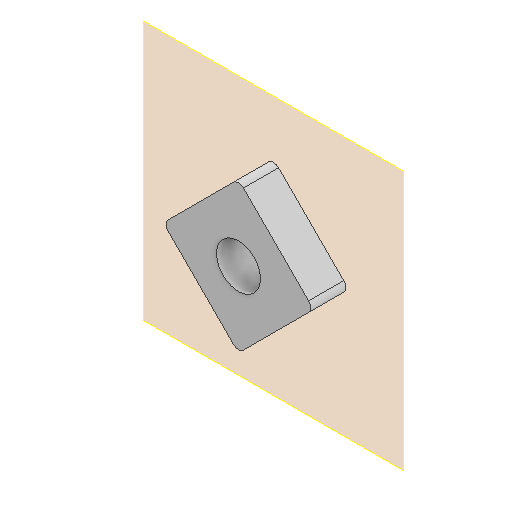
# Autodesk Inventor part: IM_Matchboxscope_lightdiffusor
Saved by Autodesk Inventor 2022 (Build 260153000, 153)
## iProperties
Created: 2023-06-16
Part Number: IM_Matchboxscope_lightdiffusor
Material: Generisch
Document SubType Name: Modeling
Designer: diederichbenedict
Density: 1 g/cm^3
Appearance: Vorgabe
Author: diederichbenedict
Autodesk Inventor part; units mm, degrees
ref_plane "YZ Plane" through (0, 0, 0) normal (1, 0, 0) x (0, 1, 0)
ref_plane "XZ Plane" through (0, 0, 0) normal (0, 1, 0) x (-1, 0, 0)
ref_plane "XY Plane" through (0, 0, 0) normal (0, 0, 1) x (1, 0, 0)
ref_plane "Arbeitsebene1" through (0, 0, 0) normal (0, 0, 1) x (1, 0, 0)
sketch "Skizze1" plane through (0, 0, 0) normal (0, 0, 1) x (1, 0, 0)
  circle A0 centre (-5.0971, -17.293) radius 1.4
  circle A1 centre (-17.4192, -5.2278) radius 1.4
  arc A2 (5.6957, 26.2674) -> (7.9686, 25.6694) centre (6.0612, 23.038) ccw
  arc A3 (5.6957, 26.2674) -> (-18.8161, -19.193) centre (0, 0) ccw
  arc A4 (-18.1702, -19.8055) -> (-18.8161, -19.193) centre (-16.2778, -17.1634) ccw
  arc A5 (-18.1702, -19.8055) -> (25.9554, 6.9811) centre (0, 0) ccw
  arc A6 (25.2463, 9.2218) -> (25.9554, 6.9811) centre (22.7119, 7.1872) ccw
  arc A7 (25.2463, 9.2218) -> (7.9686, 25.6694) centre (0, 0) ccw
  spline S0 degree 3 poles (-11.5553, -6.2972) (-11.3711, -6.4814) (-11.2247, -6.6998) (-11.0238, -7.1803) (-10.9713, -7.4379) (-10.9679, -7.9586) (-11.0171, -8.2168) (-11.2083, -8.6915) (-11.3454, -8.905) (-11.5184, -9.0874) knots 0 0 0 0 0.252225 0.252225 0.504373 0.504373 0.756494 0.756494 1 1 1 1
  line L0 (-11.5553, -6.2972) -> (-16.3497, -1.5028)
  arc A8 (-16.3497, 1.4985) -> (-16.3497, -1.5028) centre (-14.8491, -0.0022) ccw
  line L1 (-16.3497, 1.4985) -> (-1.5005, 16.3477)
  arc A9 (1.5007, 16.3477) -> (-1.5005, 16.3477) centre (0.0001, 14.8471) ccw
  line L2 (1.5007, 16.3477) -> (16.35, 1.4985)
  arc A10 (16.35, -1.5028) -> (16.35, 1.4985) centre (14.8494, -0.0022) ccw
  line L3 (16.35, -1.5028) -> (1.5007, -16.352)
  arc A11 (-1.5005, -16.352) -> (1.5007, -16.352) centre (0.0001, -14.8514) ccw
  line L4 (-1.5005, -16.352) -> (-4.7949, -13.0576)
  spline S1 degree 3 poles (-7.585, -13.0208) (-7.3961, -12.8415) (-7.1739, -12.7009) (-6.6882, -12.5128) (-6.4293, -12.4671) (-5.9087, -12.4775) (-5.6519, -12.5335) (-5.1824, -12.7372) (-4.9727, -12.8798) (-4.7949, -13.0576) knots 0 0 0 0 0.252231 0.252231 0.504388 0.504388 0.756517 0.756517 1 1 1 1
  arc A12 (-11.5184, -9.0874) -> (-7.585, -13.0208) centre (-9.4998, -11.0022) ccw
  line L5 (-4.7949, -13.0576) -> (-11.5553, -6.2972)
  line L6 (-15.9962, -1.1492) -> (-11.2017, -5.9437)
  arc A13 (-11.1557, -9.4315) -> (-7.9291, -12.658) centre (-9.4998, -11.0022) ccw
  line L7 (-4.4413, -12.7041) -> (-1.1469, -15.9985)
  arc A14 (-1.1469, -15.9985) -> (1.1472, -15.9985) centre (0.0001, -14.8514) ccw
  line L8 (1.1472, -15.9985) -> (15.9964, -1.1492)
  arc A15 (15.9964, -1.1492) -> (15.9964, 1.1449) centre (14.8494, -0.0022) ccw
  line L9 (15.9964, 1.1449) -> (1.1472, 15.9941)
  arc A16 (1.1472, 15.9941) -> (-1.1469, 15.9941) centre (0.0001, 14.8471) ccw
  line L10 (-1.1469, 15.9941) -> (-15.9962, 1.1449)
  arc A17 (-15.9962, 1.1449) -> (-15.9962, -1.1492) centre (-14.8491, -0.0022) ccw
  line L11 (-4.4414, -12.704) -> (-11.2017, -5.9437)
  circle A18 centre (0, 0) radius 5
  spline S2 degree 5 poles (-11.2017, -5.9437) (-10.656, -6.4897) (-10.3193, -7.2462) (-10.3079, -8.1062) (-10.6246, -8.8713) (-11.1557, -9.4315) knots 0 0 0 0 0 0 1 1 1 1 1 1
  spline S3 degree 5 poles (-7.9291, -12.658) (-7.3689, -12.1269) (-6.6038, -11.8103) (-5.7438, -11.8216) (-4.9873, -12.1584) (-4.4413, -12.7041) knots 0 0 0 0 0 0 1 1 1 1 1 1
  point P0 (0, 0)
  dimension "d0" = 0.5
  dimension "d1" = 10
  constraints: 14 end point, 10 point on circle, 6 centre point, 2 concentric, 2 parallel, 1 coincident, 14 other
  measures "d0" distance between parallel lines of L0 L6
  measures "d1" diameter of A18
extrude "Extrusion1" add sketch "Skizze1" along normal blind 8 contours L6 A17 L10 A16 L9 A15 L8 A14 L7 L11
